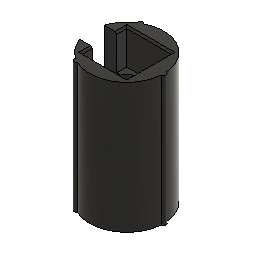
Charger_spacer_2023.04.26 (Autodesk Fusion 360 design; units mm, degrees)
Autodesk Fusion 360 part; units mm, degrees
sketch "Sketch1" plane through (0, 0, 0) normal (0, 1, 0) x (1, 0, 0) in component "SwitchSpacer"
  arc A0 (-5.8311, -8.732) -> (-5.8573, 8.7145) centre (0, 0) cw
  arc A1 (-4.6183, -9.4298) -> (-5.8311, -8.732) centre (-5.2363, -9.1011) cw
  line L0 (-20, 3.982) -> (0, 3.982)
  arc A2 (10.4756, 0.7154) -> (10.4777, -0.6839) centre (10.5, 0.0158) cw
  arc A3 (-4.6466, 9.4159) -> (10.4756, 0.7154) centre (0, 0) cw
  arc A4 (10.4777, -0.6839) -> (-4.6183, -9.4298) centre (0, 0) cw
  arc A5 (-5.8573, 8.7145) -> (-4.6466, 9.4159) centre (-5.2637, 9.0854) cw
  line L1 (-20, -4.0237) -> (-20, 3.982)
  circle A6 centre (0, 0) radius 8
  line L2 (0, 3.982) -> (0, -4.0237)
  line L3 (0, -4.0237) -> (-20, -4.0237)
  circle A7 centre (0, 0) radius 5
  circle A8 centre (0, 0) radius 4
  dimension "d8" = 10
  dimension "d9" = 8
  constraint concentric A0 A7
  constraint concentric A3 A8
  measures "d8" diameter of A7
  measures "d9" diameter of A8
extrude "Extrude8" add sketch "Sketch1" along normal blind 27 contours A0 A1 L0 A2 A3 A4 A5 A6 L3 | A0 L0 A6 L3 | L0 A6 L3 A7 | L0 A6 L3 A7 | L0 L2 L3 A7 A8 | L0 L2 L3 A7 A8 in component "SwitchSpacer"
sketch "Sketch2" plane through (0, 27, 0) normal (0, 1, 0) x (-1, 0, 0) in component "SwitchSpacer"
  circle A0 centre (0, 0) radius 4
  line L0 (6.35, 6.35) -> (-6.35, 6.35)
  line L1 (-6.35, 6.35) -> (-6.35, -6.35)
  line L2 (-6.35, -6.35) -> (6.35, -6.35)
  line L3 (6.35, -6.35) -> (6.35, 6.35)
  line L4 (6.35, 6.35) -> (-6.35, -6.35) construction
  line L5 (-6.35, 6.35) -> (6.35, -6.35) construction
  line L6 (6.35, 6.35) -> (19.35, 6.35)
  line L7 (19.35, 6.35) -> (19.35, -6.35)
  line L8 (19.35, -6.35) -> (6.35, -6.35)
  line L9 (6.35, -6.35) -> (6.35, 6.35)
  circle A1 centre (0, 0) radius 6.35
  line L10 (12.5, -3.5) -> (-12.5, -3.5)
  line L11 (-12.5, -3.5) -> (-12.5, 3.5)
  line L12 (-12.5, 3.5) -> (12.5, 3.5)
  line L13 (12.5, 3.5) -> (12.5, -3.5)
  line L14 (12.5, -3.5) -> (-12.5, 3.5) construction
  line L15 (-12.5, -3.5) -> (12.5, 3.5) construction
  arc A2 (5.8573, -8.7145) -> (5.8311, 8.732) centre (0, 0) ccw
  arc A3 (5.8311, 8.732) -> (4.6183, 9.4298) centre (5.2363, 9.1011) ccw
  arc A4 (4.6183, 9.4298) -> (-10.4777, 0.6839) centre (0, 0) ccw
  arc A5 (-10.4777, 0.6839) -> (-10.4756, -0.7154) centre (-10.5, -0.0158) ccw
  arc A6 (-10.4756, -0.7154) -> (4.6466, -9.4159) centre (0, 0) ccw
  arc A7 (4.6466, -9.4159) -> (5.8573, -8.7145) centre (5.2637, -9.0854) ccw
  circle A8 centre (0, 0) radius 4
  dimension "d18" = 12.7
  dimension "d19" = 12.7
  dimension "d20" = 13
  dimension "d21" = 12.7
  dimension "d22" = 12.7
  dimension "d27" = 25
  dimension "d28" = 7
  constraint horizontal L0
  constraint perpendicular L0 L1
  constraint parallel L0 L2
  constraint parallel L1 L3
  constraint coincident L4 A0.centre
  constraint coincident L5 A0.centre
  constraint coincident A0.centre A1.centre
  constraint horizontal L6
  constraint vertical L7
  constraint horizontal L8
  constraint vertical L9
  constraint horizontal L10
  constraint perpendicular L10 L11
  constraint parallel L10 L12
  constraint parallel L11 L13
  constraint coincident L14 A0.centre
  constraint coincident L15 A0.centre
  measures "d18" distance of L1.end L2.end
  measures "d19" distance of L0.end L1.end
  measures "d20" distance of L0.start L6.end
  measures "d21" distance of L0.start L2.end
  measures "d22" diameter of A1
  measures "d27" distance of L11.end L12.end
  measures "d28" distance of L10.end L11.end
extrude "Extrude9" cut sketch "Sketch1" along normal blind 6 contours L0 L2 L3 A7 A8 | L0 L2 L3 A7 A8 in component "SwitchSpacer"
extrude "Extrude10" add sketch "Sketch2" along normal blind 10 contours L0 L1 L6 L12 A2 A3 A4 | L3 L6 L9 L12 A2 | L1 L2 L8 L10 A2 A6 A7 | L3 L8 L9 L10 A2 | L1 L10 L12 A4 A5 A6 in component "SwitchSpacer"
extrude "Extrude11" cut sketch "Sketch2" against normal blind 17 contours A0 A1 L10 L12 A8 | A0 A1 L12 A8 | A0 A1 L10 A8 | A0 A1 L10 L12 A8 | L3 L9 A1 L12 | L3 L9 A1 L10 | L3 L9 L10 L12 A2 in component "SwitchSpacer"
fillet "Fillet1" radius 3 2 edges at (-7.5989, 10, -3.5) (-7.5989, 10, 3.5) in component "SwitchSpacer"
chamfer "Chamfer1" distance 0.5 angle 45 5 edges at (-6.35, 37, -4.925) (0, 37, -6.35) (-6.35, 37, 4.925) (0, 37, 6.35) (6.35, 37, 0) in component "SwitchSpacer"
component "SwitchSpacer" placed x (1, 0, 0) y (0, 1, 0) z (0, 0, 1) at (0, 0, 0)
